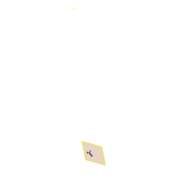
# Autodesk Inventor part: Agarre Cortadora
Saved by Autodesk Inventor 2021 (Build 250183000, 183)
## iProperties
Created: 2021-07-14
Part Number: Agarre Cortadora
Material: Generic
Document SubType Name: Modeling
Designer: maaro
Density: 1 g/cm^3
Appearance: Default
Author: maaro
Autodesk Inventor part; units mm, degrees
ref_plane "YZ Plane" through (0, 0, 0) normal (1, 0, 0) x (0, 1, 0)
ref_plane "XZ Plane" through (0, 0, 0) normal (0, 1, 0) x (-1, 0, 0)
ref_plane "XY Plane" through (0, 0, 0) normal (0, 0, 1) x (1, 0, 0)
ref_plane "Work Plane1" through (838.3238, -6744.4303, 0) normal (0, 0, 1) x (-0.969394, -0.2455104, 0)
sketch "Sketch1" plane through (838.3238, -6744.4303, 0) normal (0, 0, 1) x (-0.969394, -0.2455104, 0)
  circle A0 centre (0, 0) radius 35
  circle A1 centre (0, 0) radius 25
  arc A2 (-5.7334, 13.861) -> (-0.8591, 14.9754) centre (0, 0) ccw
  line L0 (-0.8591, 14.9754) -> (-2.9117, 23.9535)
  line L1 (-2.9117, 23.9535) -> (1.4752, 24.9564)
  arc A3 (-12.1727, 21.8363) -> (1.4752, 24.9564) centre (0, 0) ccw
  line L2 (-12.1727, 21.8363) -> (-7.7859, 22.8392)
  line L3 (-7.7859, 22.8392) -> (-5.7334, 13.861)
  point P0 (-843.1619, -6743.8271)
  dimension "d0" = 70
  dimension "d1" = 50
  constraints: 8 end point, 4 centre point, 4 point on circle, 1 coincident, 1 concentric, 14 other
  measures "d0" diameter of A0
  measures "d1" diameter of A1
extrude "Extrusion1" add sketch "Sketch1" along normal mid plane 150
sketch "Sketch2" plane through (838.3238, -6744.4303, 0) normal (0, 0, 1) x (-0.969394, -0.2455104, 0)
  point P0 (-843.1619, -6743.8271)
sketch "Sketch3" plane through (838.3238, -6744.4303, 0) normal (0, 0, 1) x (-0.969394, -0.2455104, 0)
  circle A0 centre (0, 0) radius 35 projected
  arc A1 (-11.9707, 32.8892) -> (-31.7208, 14.7916) centre (0, 0) ccw
  line L0 (0, 0) -> (-11.9707, 32.8892) construction
  line L1 (0, 0) -> (35, 0) construction
  line L2 (0, 0) -> (-31.7208, 14.7916) construction
  line L3 (-11.9707, 32.8892) -> (-31.7208, 14.7916) construction
  line L4 (-11.9707, 32.8892) -> (-147.0887, 180.3447)
  line L5 (-147.0887, 180.3447) -> (-166.8388, 162.2471)
  line L6 (-166.8388, 162.2471) -> (-31.7208, 14.7916)
  line L7 (-140.074, 152.864) -> (-72.515, 79.1362) construction
  line L8 (-143.7604, 149.486) -> (-76.2014, 75.7583)
  line L9 (-68.8286, 82.5142) -> (-136.3876, 156.2419)
  arc A2 (-136.3876, 156.2419) -> (-143.7604, 149.486) centre (-140.074, 152.864) ccw
  arc A3 (-76.2014, 75.7583) -> (-68.8286, 82.5142) centre (-72.515, 79.1362) ccw
  point P0 (-843.1619, -6743.8271)
  point P1 (-106.2945, 116.0001)
  point P2 (-156.9638, 171.2959)
  dimension "d4" = 35
  dimension "d5" = 110
  dimension "d6" = 45
  dimension "d7" = 200
  dimension "d8" = 200
  dimension "d9" = 100
  dimension "d10" = 10
  dimension "d11" = 25
  constraints: 22 end point, 8 point on circle, 4 tangent, 3 centre point, 3 perpendicular, 2 midpoint, 1 equal length, 1 horizontal, 1 parallel, 1 point on line
  measures "d4" radius of A1
  measures "d5" angle of L1 L0
  measures "d6" angle of L0 L2
  measures "d7" distance of L0.end L4.end
  measures "d8" distance of L5.end L2.end
  measures "d9" distance of L7.start L7.end
  measures "d10" diameter of A3
  measures "d11" distance from line of L7.start L5
extrude "Extrusion2" add sketch "Sketch3" along normal mid plane 40 contours A0 L6 L5 L4
body "Solid1"
